Autodesk Fusion 360 part; units mm, degrees
note: some values were not read from the file. Chosen so that the rebuilt part matches the saved one: which face or edge a step refers to. Set by a fixed rule: which sketch regions a step uses.
(part 6 of 7)
  arc A131 (-37.243, 7.9658) -> (-36.8156, 8.2763) centre (-37.2058, 8.364) ccw
  spline S129 degree 3 poles (-38.191, 7.9821) (-37.7562, 8.0001) (-37.442, 7.9843) (-37.243, 7.9658) knots 0 0 0 0 1 1 1 1
  spline S130 degree 3 poles (-41.6177, 7.3659) (-40.1262, 7.8053) (-38.9736, 7.9493) (-38.191, 7.9821) knots 0 0 0 0 1 1 1 1
  arc A132 (-41.6177, 7.3659) -> (-41.857, 5.8552) centre (0, 0) ccw
  spline S131 degree 3 poles (-38.7884, 4.2102) (-39.5225, 4.4833) (-40.5743, 4.9764) (-41.857, 5.8552) knots 0 0 0 0 1 1 1 1
  spline S132 degree 3 poles (-37.8817, 3.9328) (-38.0767, 3.9767) (-38.3805, 4.0588) (-38.7884, 4.2102) knots 0 0 0 0 1 1 1 1
  arc A133 (-37.5712, 3.5054) -> (-37.8817, 3.9328) centre (-37.9695, 3.5426) ccw
  arc A134 (-37.5712, 3.5054) -> (-37.657, 2.4152) centre (0, 0) ccw
  arc A135 (-38.0306, 2.0416) -> (-37.657, 2.4152) centre (-38.0562, 2.4408) ccw
  spline S133 degree 3 poles (-38.9695, 1.9094) (-38.5429, 1.9952) (-38.23, 2.0288) (-38.0306, 2.0416) knots 0 0 0 0 1 1 1 1
  spline S134 degree 3 poles (-42.2576, 0.7648) (-40.8532, 1.4321) (-39.7373, 1.7546) (-38.9695, 1.9094) knots 0 0 0 0 1 1 1 1
  arc A136 (-42.2576, 0.7648) -> (-42.2576, -0.7648) centre (0, 0) ccw
  spline S135 degree 3 poles (-38.9695, -1.9094) (-39.7373, -1.7546) (-40.8532, -1.4321) (-42.2576, -0.7648) knots 0 0 0 0 1 1 1 1
  spline S136 degree 3 poles (-38.0306, -2.0416) (-38.23, -2.0288) (-38.5429, -1.9952) (-38.9695, -1.9094) knots 0 0 0 0 1 1 1 1
  arc A137 (-37.657, -2.4152) -> (-38.0306, -2.0416) centre (-38.0562, -2.4408) ccw
  arc A138 (-37.657, -2.4152) -> (-37.5712, -3.5054) centre (0, 0) ccw
  arc A139 (-37.8817, -3.9328) -> (-37.5712, -3.5054) centre (-37.9695, -3.5426) ccw
  spline S137 degree 3 poles (-38.7884, -4.2102) (-38.3805, -4.0588) (-38.0767, -3.9767) (-37.8817, -3.9328) knots 0 0 0 0 1 1 1 1
  spline S138 degree 3 poles (-41.857, -5.8552) (-40.5743, -4.9764) (-39.5225, -4.4833) (-38.7884, -4.2102) knots 0 0 0 0 1 1 1 1
  arc A140 (-41.857, -5.8552) -> (-41.6177, -7.3659) centre (0, 0) ccw
  spline S139 degree 3 poles (-38.191, -7.9821) (-38.9736, -7.9493) (-40.1262, -7.8053) (-41.6177, -7.3659) knots 0 0 0 0 1 1 1 1
  spline S140 degree 3 poles (-37.243, -7.9658) (-37.442, -7.9843) (-37.7562, -8.0001) (-38.191, -7.9821) knots 0 0 0 0 1 1 1 1
  arc A141 (-36.8156, -8.2763) -> (-37.243, -7.9658) centre (-37.2058, -8.364) ccw
  arc A142 (-36.8156, -8.2763) -> (-36.5603, -9.3397) centre (0, 0) ccw
  arc A143 (-36.8001, -9.8104) -> (-36.5603, -9.3397) centre (-36.9478, -9.4387) ccw
  spline S141 degree 3 poles (-37.6523, -10.2263) (-37.273, -10.0128) (-36.9859, -9.8842) (-36.8001, -9.8104) knots 0 0 0 0 1 1 1 1
  spline S142 degree 3 poles (-40.4257, -12.331) (-39.2962, -11.2623) (-38.3346, -10.6107) (-37.6523, -10.2263) knots 0 0 0 0 1 1 1 1
  arc A144 (-40.4257, -12.331) -> (-39.953, -13.7857) centre (0, 0) ccw
  spline S143 degree 3 poles (-36.4722, -13.8582) (-37.2502, -13.9482) (-38.4112, -13.9863) (-39.953, -13.7857) knots 0 0 0 0 1 1 1 1
  spline S144 degree 3 poles (-35.5383, -13.6938) (-35.732, -13.7432) (-36.0399, -13.808) (-36.4722, -13.8582) knots 0 0 0 0 1 1 1 1
  arc A145 (-35.0676, -13.9336) -> (-35.5383, -13.6938) centre (-35.4393, -14.0813) ccw
  arc A146 (-35.0676, -13.9336) -> (-34.6491, -14.944) centre (0, 0) ccw
  arc A147 (-34.8123, -15.4464) -> (-34.6491, -14.944) centre (-35.0164, -15.1024) ccw
  spline S145 degree 3 poles (-35.5889, -15.9905) (-35.2478, -15.7204) (-34.9843, -15.5484) (-34.8123, -15.4464) knots 0 0 0 0 1 1 1 1
  spline S146 degree 3 poles (-37.999, -18.5031) (-37.0506, -17.271) (-36.2028, -16.477) (-35.5889, -15.9905) knots 0 0 0 0 1 1 1 1
  arc A148 (-37.999, -18.5031) -> (-37.3046, -19.866) centre (0, 0) ccw
  spline S147 degree 3 poles (-33.8552, -19.3931) (-34.6096, -19.6037) (-35.7503, -19.823) (-37.3046, -19.866) knots 0 0 0 0 1 1 1 1
  spline S148 degree 3 poles (-32.9586, -19.0846) (-33.1422, -19.1638) (-33.4362, -19.2759) (-33.8552, -19.3931) knots 0 0 0 0 1 1 1 1
  arc A149 (-32.4562, -19.2479) -> (-32.9586, -19.0846) centre (-32.8002, -19.4519) ccw
  arc A150 (-32.4562, -19.2479) -> (-31.8848, -20.1803) centre (0, 0) ccw
  arc A151 (-31.9674, -20.7021) -> (-31.8848, -20.1803) centre (-32.2228, -20.3942) ccw
  spline S149 degree 3 poles (-32.6493, -21.3609) (-32.3546, -21.0408) (-32.1213, -20.8297) (-31.9674, -20.7021) knots 0 0 0 0 1 1 1 1
  spline S150 degree 3 poles (-34.6367, -24.2197) (-33.8927, -22.8543) (-33.1795, -21.9375) (-32.6493, -21.3609) knots 0 0 0 0 1 1 1 1
  arc A152 (-34.6367, -24.2197) -> (-33.7376, -25.4571) centre (0, 0) ccw
  spline S151 degree 3 poles (-30.4047, -24.4505) (-31.1168, -24.7765) (-32.2092, -25.1715) (-33.7376, -25.4571) knots 0 0 0 0 1 1 1 1
  spline S152 degree 3 poles (-29.5673, -24.0055) (-29.7363, -24.1124) (-30.0091, -24.2691) (-30.4047, -24.4505) knots 0 0 0 0 1 1 1 1
  arc A153 (-29.0455, -24.0882) -> (-29.5673, -24.0055) centre (-29.3534, -24.3435) ccw
  arc A154 (-29.0455, -24.0882) -> (-28.3353, -24.9197) centre (0, 0) ccw
  arc A155 (-28.3353, -25.448) -> (-28.3353, -24.9197) centre (-28.6357, -25.1839) ccw
  spline S153 degree 3 poles (-28.9058, -26.2054) (-28.6648, -25.8431) (-28.4673, -25.5981) (-28.3353, -25.448) knots 0 0 0 0 1 1 1 1
  spline S154 degree 3 poles (-30.4214, -29.3399) (-29.9002, -27.8749) (-29.3392, -26.8578) (-28.9058, -26.2054) knots 0 0 0 0 1 1 1 1
  arc A156 (-30.4214, -29.3399) -> (-29.3399, -30.4214) centre (0, 0) ccw
  spline S155 degree 3 poles (-26.2054, -28.9058) (-26.8578, -29.3392) (-27.8749, -29.9002) (-29.3399, -30.4214) knots 0 0 0 0 1 1 1 1
  spline S156 degree 3 poles (-25.448, -28.3353) (-25.5981, -28.4673) (-25.8431, -28.6648) (-26.2054, -28.9058) knots 0 0 0 0 1 1 1 1
  arc A157 (-24.9197, -28.3353) -> (-25.448, -28.3353) centre (-25.1839, -28.6357) ccw
  arc A158 (-24.9197, -28.3353) -> (-24.0882, -29.0455) centre (0, 0) ccw
  arc A159 (-24.0055, -29.5673) -> (-24.0882, -29.0455) centre (-24.3435, -29.3534) ccw
  spline S157 degree 3 poles (-24.4505, -30.4047) (-24.2691, -30.0091) (-24.1124, -29.7363) (-24.0055, -29.5673) knots 0 0 0 0 1 1 1 1
  spline S158 degree 3 poles (-25.4571, -33.7376) (-25.1715, -32.2092) (-24.7765, -31.1168) (-24.4505, -30.4047) knots 0 0 0 0 1 1 1 1
  arc A160 (-25.4571, -33.7376) -> (-24.2197, -34.6367) centre (0, 0) ccw
  spline S159 degree 3 poles (-21.3609, -32.6493) (-21.9375, -33.1795) (-22.8543, -33.8927) (-24.2197, -34.6367) knots 0 0 0 0 1 1 1 1
  circle A161 centre (0, 0) radius 3.85
extrude "Extrude2'''" add sketch "Sketch21" along normal blind -8 and the other way blind -40 separate body contours A0 A161 makes body 8 in component "Spur Gear (40 teeth)"
sketch "Sketch22" plane through (0, 20, 0) normal (0, 1, 0) x (-1, 0, 0)
  circle A0 centre (0, 0) radius 3.85
  circle A1 centre (58.2177, 14.5153) radius 5.25
  circle A2 centre (-41.6795, 43.1604) radius 5.25
  circle A3 centre (-16.5382, -57.6757) radius 5.25
  line L0 (-22.7416, -43.0299) -> (-27.9212, -61.0931)
  arc A4 (-27.9212, -61.0931) -> (-27.7213, -63.2604) centre (-25.0374, -61.9201) ccw
  arc A5 (-27.7213, -63.2604) -> (-10.0139, -68.3379) centre (-16.5382, -57.6757) ccw
  arc A6 (-10.0139, -68.3379) -> (-8.6959, -66.6059) centre (-11.5797, -65.779) ccw
  line L1 (-8.6959, -66.6059) -> (-3.5164, -48.5426)
  arc A7 (48.6358, 1.8201) -> (-3.5164, -48.5426) centre (66.1751, -68.5263) ccw
  line L2 (48.6358, 1.8201) -> (66.8688, 6.3661)
  arc A8 (66.8688, 6.3661) -> (68.6458, 7.6228) centre (66.143, 9.277) ccw
  arc A9 (68.6458, 7.6228) -> (64.1893, 25.4967) centre (58.2177, 14.5153) ccw
  arc A10 (64.1893, 25.4967) -> (62.0304, 25.772) centre (62.7561, 22.8612) ccw
  line L3 (62.0304, 25.772) -> (43.7973, 21.226)
  arc A11 (-25.8942, 41.2097) -> (43.7973, 21.226) centre (26.258, 91.5725) ccw
  line L4 (-25.8942, 41.2097) -> (-38.9476, 54.727)
  arc A12 (-38.9476, 54.727) -> (-40.9244, 55.6376) centre (-41.1056, 52.643) ccw
  arc A13 (-40.9244, 55.6376) -> (-54.1754, 42.8412) centre (-41.6795, 43.1604) ccw
  arc A14 (-54.1754, 42.8412) -> (-53.3344, 40.8338) centre (-51.1764, 42.9178) ccw
  line L5 (-53.3344, 40.8338) -> (-40.2809, 27.3166)
  arc A15 (-22.7416, -43.0299) -> (-40.2809, 27.3166) centre (-92.4331, -23.0462) ccw
  circle A16 centre (0, 0) radius 3.85
extrude "Extrude3'" add sketch "Sketch22" along normal blind 40 and the other way blind 8 contours A0 A16 bodies 6 in component "Component''"
sketch "Sketch23" plane through (0, 8, 0) normal (0, 1, 0) x (-1, 0, 0)
  spline S0 degree 3 poles (-79.7947, 19.9812) (-78.771, 20.1522) (-77.8517, 20.2559) (-77.0419, 20.3133) knots 0 0 0 0 1 1 1 1
  spline S1 degree 3 poles (-77.0419, 20.3133) (-76.8232, 20.3288) (-76.6126, 20.341) (-76.41, 20.3501) knots 0 0 0 0 1 1 1 1
  arc A0 (-76.41, 20.3501) -> (-76.0422, 20.6449) centre (-76.4282, 20.7497) ccw
  arc A1 (-75.6235, 22.1292) -> (-76.0422, 20.6449) centre (0, 0) ccw
  arc A2 (-75.6235, 22.1292) -> (-75.7832, 22.5728) centre (-76.0074, 22.2416) ccw
  spline S2 degree 3 poles (-75.7832, 22.5728) (-75.9511, 22.6864) (-76.1243, 22.8068) (-76.3027, 22.9343) knots 0 0 0 0 1 1 1 1
  spline S3 degree 3 poles (-76.3027, 22.9343) (-76.9632, 23.4064) (-77.6928, 23.9752) (-78.4763, 24.6558) knots 0 0 0 0 1 1 1 1
  arc A3 (-77.981, 26.1802) -> (-78.4763, 24.6558) centre (0, 0) ccw
  spline S4 degree 3 poles (-77.981, 26.1802) (-76.9471, 26.2704) (-76.0225, 26.3016) (-75.2107, 26.2953) knots 0 0 0 0 1 1 1 1
  spline S5 degree 3 poles (-75.2107, 26.2953) (-74.9914, 26.2937) (-74.7805, 26.2892) (-74.5778, 26.2825) knots 0 0 0 0 1 1 1 1
  arc A4 (-74.5778, 26.2825) -> (-74.188, 26.5475) centre (-74.5646, 26.6822) ccw
  arc A5 (-73.6542, 27.9944) -> (-74.188, 26.5475) centre (0, 0) ccw
  arc A6 (-73.6542, 27.9944) -> (-73.7785, 28.4491) centre (-74.0281, 28.1365) ccw
  spline S6 degree 3 poles (-73.7785, 28.4491) (-73.937, 28.5755) (-74.1003, 28.7092) (-74.2681, 28.8503) knots 0 0 0 0 1 1 1 1
  spline S7 degree 3 poles (-74.2681, 28.8503) (-74.8895, 29.3727) (-75.5723, 29.997) (-76.2999, 30.737) knots 0 0 0 0 1 1 1 1
  arc A7 (-75.6865, 32.2178) -> (-76.2999, 30.737) centre (0, 0) ccw
  spline S8 degree 3 poles (-75.6865, 32.2178) (-74.6487, 32.2266) (-73.7245, 32.1852) (-72.9157, 32.1152) knots 0 0 0 0 1 1 1 1
  spline S9 degree 3 poles (-72.9157, 32.1152) (-72.6972, 32.0964) (-72.4873, 32.0754) (-72.2858, 32.0528) knots 0 0 0 0 1 1 1 1
  arc A8 (-72.2858, 32.0528) -> (-71.8764, 32.2864) centre (-72.2413, 32.4503) ccw
  arc A9 (-71.2307, 33.6869) -> (-71.8764, 32.2864) centre (0, 0) ccw
  arc A10 (-71.2307, 33.6869) -> (-71.319, 34.15) centre (-71.5923, 33.8579) ccw
  spline S10 degree 3 poles (-71.319, 34.15) (-71.4671, 34.2885) (-71.6193, 34.4345) (-71.7756, 34.5883) knots 0 0 0 0 1 1 1 1
  spline S11 degree 3 poles (-71.7756, 34.5883) (-72.3541, 35.1579) (-72.9858, 35.8338) (-73.6531, 36.6287) knots 0 0 0 0 1 1 1 1
  arc A11 (-72.9254, 38.0568) -> (-73.6531, 36.6287) centre (0, 0) ccw
  spline S12 degree 3 poles (-72.9254, 38.0568) (-71.8901, 37.9841) (-70.972, 37.8704) (-70.1712, 37.7371) knots 0 0 0 0 1 1 1 1
  spline S13 degree 3 poles (-70.1712, 37.7371) (-69.9549, 37.7012) (-69.7473, 37.6638) (-69.5482, 37.6254) knots 0 0 0 0 1 1 1 1
  arc A12 (-69.5482, 37.6254) -> (-69.1217, 37.8262) centre (-69.4726, 38.0182) ccw
  arc A13 (-68.3681, 39.1718) -> (-69.1217, 37.8262) centre (0, 0) ccw
  arc A14 (-68.3681, 39.1718) -> (-68.4198, 39.6403) centre (-68.7152, 39.3706) ccw
  spline S14 degree 3 poles (-68.4198, 39.6403) (-68.5565, 39.79) (-68.6969, 39.9475) (-68.8406, 40.1132) knots 0 0 0 0 1 1 1 1
  spline S15 degree 3 poles (-68.8406, 40.1132) (-69.3726, 40.7264) (-69.9493, 41.4498) (-70.5522, 42.2945) knots 0 0 0 0 1 1 1 1
  arc A15 (-69.7147, 43.6612) -> (-70.5522, 42.2945) centre (0, 0) ccw
  spline S16 degree 3 poles (-69.7147, 43.6612) (-68.6883, 43.5075) (-67.7819, 43.322) (-66.9941, 43.1264) knots 0 0 0 0 1 1 1 1
  spline S17 degree 3 poles (-66.9941, 43.1264) (-66.7812, 43.0736) (-66.5772, 43.02) (-66.3817, 42.9661) knots 0 0 0 0 1 1 1 1
  arc A16 (-66.3817, 42.9661) -> (-65.9408, 43.1328) centre (-66.2755, 43.3518) ccw
  arc A17 (-65.084, 44.4151) -> (-65.9408, 43.1328) centre (0, 0) ccw
  arc A18 (-65.084, 44.4151) -> (-65.0987, 44.8863) centre (-65.4144, 44.6406) ccw
  spline S18 degree 3 poles (-65.0987, 44.8863) (-65.2233, 45.0463) (-65.3508, 45.2143) (-65.4811, 45.3907) knots 0 0 0 0 1 1 1 1
  spline S19 degree 3 poles (-65.4811, 45.3907) (-65.9633, 46.0437) (-66.4815, 46.8101) (-67.0163, 47.6996) knots 0 0 0 0 1 1 1 1
  arc A19 (-66.0742, 48.9963) -> (-67.0163, 47.6996) centre (0, 0) ccw
  spline S20 degree 3 poles (-66.0742, 48.9963) (-65.063, 48.7626) (-64.174, 48.5066) (-63.4039, 48.2497) knots 0 0 0 0 1 1 1 1
  spline S21 degree 3 poles (-63.4039, 48.2497) (-63.1959, 48.1804) (-62.9966, 48.111) (-62.806, 48.0419) knots 0 0 0 0 1 1 1 1
  arc A20 (-62.806, 48.0419) -> (-62.3533, 48.1735) centre (-62.6699, 48.418) ccw
  arc A21 (-61.3986, 49.3846) -> (-62.3533, 48.1735) centre (0, 0) ccw
  arc A22 (-61.3986, 49.3846) -> (-61.3763, 49.8555) centre (-61.7102, 49.6353) ccw
  spline S22 degree 3 poles (-61.3763, 49.8555) (-61.4879, 50.0247) (-61.6019, 50.2023) (-61.7179, 50.3883) knots 0 0 0 0 1 1 1 1
  spline S23 degree 3 poles (-61.7179, 50.3883) (-62.1475, 51.0772) (-62.6039, 51.8819) (-63.0673, 52.8106) knots 0 0 0 0 1 1 1 1
  arc A23 (-62.0263, 54.0294) -> (-63.0673, 52.8106) centre (0, 0) ccw
  spline S24 degree 3 poles (-62.0263, 54.0294) (-61.0366, 53.717) (-60.1704, 53.3921) (-59.4228, 53.0756) knots 0 0 0 0 1 1 1 1
  spline S25 degree 3 poles (-59.4228, 53.0756) (-59.2209, 52.9901) (-59.0277, 52.9053) (-58.8431, 52.8215) knots 0 0 0 0 1 1 1 1
  arc A24 (-58.8431, 52.8215) -> (-58.3815, 52.9172) centre (-58.6778, 53.1858) ccw
  arc A25 (-57.3346, 54.0497) -> (-58.3815, 52.9172) centre (0, 0) ccw
  arc A26 (-57.3346, 54.0497) -> (-57.2755, 54.5174) centre (-57.6257, 54.324) ccw
  spline S26 degree 3 poles (-57.2755, 54.5174) (-57.3735, 54.6948) (-57.4732, 54.8807) (-57.5742, 55.0753) knots 0 0 0 0 1 1 1 1
  spline S27 degree 3 poles (-57.5742, 55.0753) (-57.9484, 55.7958) (-58.3403, 56.6338) (-58.7294, 57.596) knots 0 0 0 0 1 1 1 1
  arc A27 (-57.596, 58.7294) -> (-58.7294, 57.596) centre (0, 0) ccw
  spline S28 degree 3 poles (-57.596, 58.7294) (-56.6338, 58.3403) (-55.7958, 57.9484) (-55.0753, 57.5742) knots 0 0 0 0 1 1 1 1
  spline S29 degree 3 poles (-55.0753, 57.5742) (-54.8807, 57.4732) (-54.6948, 57.3735) (-54.5174, 57.2755) knots 0 0 0 0 1 1 1 1
  arc A28 (-54.5174, 57.2755) -> (-54.0497, 57.3346) centre (-54.324, 57.6257) ccw
  arc A29 (-52.9172, 58.3815) -> (-54.0497, 57.3346) centre (0, 0) ccw
  arc A30 (-52.9172, 58.3815) -> (-52.8215, 58.8431) centre (-53.1858, 58.6778) ccw
  spline S30 degree 3 poles (-52.8215, 58.8431) (-52.9053, 59.0277) (-52.9901, 59.2209) (-53.0756, 59.4228) knots 0 0 0 0 1 1 1 1
  spline S31 degree 3 poles (-53.0756, 59.4228) (-53.3921, 60.1704) (-53.717, 61.0366) (-54.0294, 62.0263) knots 0 0 0 0 1 1 1 1
  arc A31 (-52.8106, 63.0673) -> (-54.0294, 62.0263) centre (0, 0) ccw
  spline S32 degree 3 poles (-52.8106, 63.0673) (-51.8819, 62.6039) (-51.0772, 62.1475) (-50.3883, 61.7179) knots 0 0 0 0 1 1 1 1
  spline S33 degree 3 poles (-50.3883, 61.7179) (-50.2023, 61.6019) (-50.0247, 61.4879) (-49.8555, 61.3763) knots 0 0 0 0 1 1 1 1
  arc A32 (-49.8555, 61.3763) -> (-49.3846, 61.3986) centre (-49.6353, 61.7102) ccw
  arc A33 (-48.1735, 62.3533) -> (-49.3846, 61.3986) centre (0, 0) ccw
  arc A34 (-48.1735, 62.3533) -> (-48.0419, 62.806) centre (-48.418, 62.6699) ccw
  spline S34 degree 3 poles (-48.0419, 62.806) (-48.111, 62.9966) (-48.1804, 63.1959) (-48.2497, 63.4039) knots 0 0 0 0 1 1 1 1
  spline S35 degree 3 poles (-48.2497, 63.4039) (-48.5066, 64.174) (-48.7626, 65.063) (-48.9963, 66.0742) knots 0 0 0 0 1 1 1 1
  arc A35 (-47.6996, 67.0163) -> (-48.9963, 66.0742) centre (0, 0) ccw
  spline S36 degree 3 poles (-47.6996, 67.0163) (-46.8101, 66.4815) (-46.0437, 65.9633) (-45.3907, 65.4811) knots 0 0 0 0 1 1 1 1
  spline S37 degree 3 poles (-45.3907, 65.4811) (-45.2143, 65.3508) (-45.0463, 65.2233) (-44.8863, 65.0987) knots 0 0 0 0 1 1 1 1
  arc A36 (-44.8863, 65.0987) -> (-44.4151, 65.084) centre (-44.6406, 65.4144) ccw
  arc A37 (-43.1328, 65.9408) -> (-44.4151, 65.084) centre (0, 0) ccw
  arc A38 (-43.1328, 65.9408) -> (-42.9661, 66.3817) centre (-43.3518, 66.2755) ccw
  spline S38 degree 3 poles (-42.9661, 66.3817) (-43.02, 66.5772) (-43.0736, 66.7812) (-43.1264, 66.9941) knots 0 0 0 0 1 1 1 1
  spline S39 degree 3 poles (-43.1264, 66.9941) (-43.322, 67.7819) (-43.5075, 68.6883) (-43.6612, 69.7147) knots 0 0 0 0 1 1 1 1
  arc A39 (-42.2945, 70.5522) -> (-43.6612, 69.7147) centre (0, 0) ccw
  spline S40 degree 3 poles (-42.2945, 70.5522) (-41.4498, 69.9493) (-40.7264, 69.3726) (-40.1132, 68.8406) knots 0 0 0 0 1 1 1 1
  spline S41 degree 3 poles (-40.1132, 68.8406) (-39.9475, 68.6969) (-39.79, 68.5565) (-39.6403, 68.4198) knots 0 0 0 0 1 1 1 1
  arc A40 (-39.6403, 68.4198) -> (-39.1718, 68.3681) centre (-39.3706, 68.7152) ccw
  arc A41 (-37.8262, 69.1217) -> (-39.1718, 68.3681) centre (0, 0) ccw
  arc A42 (-37.8262, 69.1217) -> (-37.6254, 69.5482) centre (-38.0182, 69.4726) ccw
  spline S42 degree 3 poles (-37.6254, 69.5482) (-37.6638, 69.7473) (-37.7012, 69.9549) (-37.7371, 70.1712) knots 0 0 0 0 1 1 1 1
  spline S43 degree 3 poles (-37.7371, 70.1712) (-37.8704, 70.972) (-37.9841, 71.8901) (-38.0568, 72.9254) knots 0 0 0 0 1 1 1 1
  arc A43 (-36.6287, 73.6531) -> (-38.0568, 72.9254) centre (0, 0) ccw
  spline S44 degree 3 poles (-36.6287, 73.6531) (-35.8338, 72.9858) (-35.1579, 72.3541) (-34.5883, 71.7756) knots 0 0 0 0 1 1 1 1
  spline S45 degree 3 poles (-34.5883, 71.7756) (-34.4345, 71.6193) (-34.2885, 71.4671) (-34.15, 71.319) knots 0 0 0 0 1 1 1 1
  arc A44 (-34.15, 71.319) -> (-33.6869, 71.2307) centre (-33.8579, 71.5923) ccw
  arc A45 (-32.2864, 71.8764) -> (-33.6869, 71.2307) centre (0, 0) ccw
  arc A46 (-32.2864, 71.8764) -> (-32.0528, 72.2858) centre (-32.4503, 72.2413) ccw
  spline S46 degree 3 poles (-32.0528, 72.2858) (-32.0754, 72.4873) (-32.0964, 72.6972) (-32.1152, 72.9157) knots 0 0 0 0 1 1 1 1
  spline S47 degree 3 poles (-32.1152, 72.9157) (-32.1852, 73.7245) (-32.2266, 74.6487) (-32.2178, 75.6865) knots 0 0 0 0 1 1 1 1
  arc A47 (-30.737, 76.2999) -> (-32.2178, 75.6865) centre (0, 0) ccw
  spline S48 degree 3 poles (-30.737, 76.2999) (-29.997, 75.5723) (-29.3727, 74.8895) (-28.8503, 74.2681) knots 0 0 0 0 1 1 1 1
  spline S49 degree 3 poles (-28.8503, 74.2681) (-28.7092, 74.1003) (-28.5755, 73.937) (-28.4491, 73.7785) knots 0 0 0 0 1 1 1 1
  arc A48 (-28.4491, 73.7785) -> (-27.9944, 73.6542) centre (-28.1365, 74.0281) ccw
  arc A49 (-26.5475, 74.188) -> (-27.9944, 73.6542) centre (0, 0) ccw
  arc A50 (-26.5475, 74.188) -> (-26.2825, 74.5778) centre (-26.6822, 74.5646) ccw
  spline S50 degree 3 poles (-26.2825, 74.5778) (-26.2892, 74.7805) (-26.2937, 74.9914) (-26.2953, 75.2107) knots 0 0 0 0 1 1 1 1
  spline S51 degree 3 poles (-26.2953, 75.2107) (-26.3016, 76.0225) (-26.2704, 76.9471) (-26.1802, 77.981) knots 0 0 0 0 1 1 1 1
  arc A51 (-24.6558, 78.4763) -> (-26.1802, 77.981) centre (0, 0) ccw
  spline S52 degree 3 poles (-24.6558, 78.4763) (-23.9752, 77.6928) (-23.4064, 76.9632) (-22.9343, 76.3027) knots 0 0 0 0 1 1 1 1
  spline S53 degree 3 poles (-22.9343, 76.3027) (-22.8068, 76.1243) (-22.6864, 75.9511) (-22.5728, 75.7832) knots 0 0 0 0 1 1 1 1
  arc A52 (-22.5728, 75.7832) -> (-22.1292, 75.6235) centre (-22.2416, 76.0074) ccw
  arc A53 (-20.6449, 76.0422) -> (-22.1292, 75.6235) centre (0, 0) ccw
  arc A54 (-20.6449, 76.0422) -> (-20.3501, 76.41) centre (-20.7497, 76.4282) ccw
  spline S54 degree 3 poles (-20.3501, 76.41) (-20.341, 76.6126) (-20.3288, 76.8232) (-20.3133, 77.0419) knots 0 0 0 0 1 1 1 1
  spline S55 degree 3 poles (-20.3133, 77.0419) (-20.2559, 77.8517) (-20.1522, 78.771) (-19.9812, 79.7947) knots 0 0 0 0 1 1 1 1
  arc A55 (-18.4227, 80.1689) -> (-19.9812, 79.7947) centre (0, 0) ccw
  spline S56 degree 3 poles (-18.4227, 80.1689) (-17.8055, 79.3344) (-17.2958, 78.5624) (-16.877, 77.8669) knots 0 0 0 0 1 1 1 1
  spline S57 degree 3 poles (-16.877, 77.8669) (-16.7639, 77.6791) (-16.6574, 77.4969) (-16.5573, 77.3206) knots 0 0 0 0 1 1 1 1
  arc A56 (-16.5573, 77.3206) -> (-16.1277, 77.1267) centre (-16.2095, 77.5182) ccw
  arc A57 (-14.6151, 77.4275) -> (-16.1277, 77.1267) centre (0, 0) ccw
  arc A58 (-14.6151, 77.4275) -> (-14.2923, 77.7712) centre (-14.6893, 77.8206) ccw
  spline S58 degree 3 poles (-14.2923, 77.7712) (-14.2673, 77.9723) (-14.2387, 78.1814) (-14.2061, 78.3982) knots 0 0 0 0 1 1 1 1
  spline S59 degree 3 poles (-14.2061, 78.3982) (-14.0853, 79.201) (-13.9098, 80.1093) (-13.659, 81.1164) knots 0 0 0 0 1 1 1 1
  arc A59 (-12.0759, 81.3672) -> (-13.659, 81.1164) centre (0, 0) ccw
  spline S60 degree 3 poles (-12.0759, 81.3672) (-11.5261, 80.4868) (-11.0785, 79.6772) (-10.7156, 78.951) knots 0 0 0 0 1 1 1 1
  spline S61 degree 3 poles (-10.7156, 78.951) (-10.6176, 78.7549) (-10.5258, 78.5649) (-10.4398, 78.3813) knots 0 0 0 0 1 1 1 1
  arc A60 (-10.4398, 78.3813) -> (-10.0267, 78.1543) centre (-10.0776, 78.551) ccw
  arc A61 (-8.4951, 78.3355) -> (-10.0267, 78.1543) centre (0, 0) ccw
  arc A62 (-8.4951, 78.3355) -> (-8.1464, 78.6528) centre (-8.5383, 78.7332) ccw
  spline S62 degree 3 poles (-8.1464, 78.6528) (-8.1057, 78.8514) (-8.0608, 79.0575) (-8.0112, 79.2711) knots 0 0 0 0 1 1 1 1
  spline S63 degree 3 poles (-8.0112, 79.2711) (-7.8278, 80.0619) (-7.5816, 80.9537) (-7.2526, 81.938) knots 0 0 0 0 1 1 1 1
  arc A63 (-5.6547, 82.0638) -> (-7.2526, 81.938) centre (0, 0) ccw
  spline S64 degree 3 poles (-5.6547, 82.0638) (-5.1757, 81.1431) (-4.793, 80.3008) (-4.4881, 79.5484) knots 0 0 0 0 1 1 1 1
  spline S65 degree 3 poles (-4.4881, 79.5484) (-4.4058, 79.3452) (-4.3292, 79.1486) (-4.2579, 78.9588) knots 0 0 0 0 1 1 1 1
  arc A64 (-4.2579, 78.9588) -> (-3.8638, 78.7) centre (-3.8835, 79.0995) ccw
  arc A65 (-2.3228, 78.7606) -> (-3.8638, 78.7) centre (0, 0) ccw
  arc A66 (-2.3228, 78.7606) -> (-1.9503, 79.0495) centre (-2.3346, 79.1604) ccw
  spline S66 degree 3 poles (-1.9503, 79.0495) (-1.8941, 79.2443) (-1.8331, 79.4462) (-1.767, 79.6553) knots 0 0 0 0 1 1 1 1
  spline S67 degree 3 poles (-1.767, 79.6553) (-1.5221, 80.4293) (-1.2067, 81.299) (-0.8014, 82.2545) knots 0 0 0 0 1 1 1 1
  arc A67 (0.8014, 82.2545) -> (-0.8014, 82.2545) centre (0, 0) ccw
  spline S68 degree 3 poles (0.8014, 82.2545) (1.2067, 81.299) (1.5221, 80.4293) (1.767, 79.6553) knots 0 0 0 0 1 1 1 1
  spline S69 degree 3 poles (1.767, 79.6553) (1.8331, 79.4462) (1.8941, 79.2443) (1.9503, 79.0495) knots 0 0 0 0 1 1 1 1
  arc A68 (1.9503, 79.0495) -> (2.3228, 78.7606) centre (2.3346, 79.1604) ccw
  arc A69 (3.8638, 78.7) -> (2.3228, 78.7606) centre (0, 0) ccw
  arc A70 (3.8638, 78.7) -> (4.2579, 78.9588) centre (3.8835, 79.0995) ccw
  spline S70 degree 3 poles (4.2579, 78.9588) (4.3292, 79.1486) (4.4058, 79.3452) (4.4881, 79.5484) knots 0 0 0 0 1 1 1 1
  spline S71 degree 3 poles (4.4881, 79.5484) (4.793, 80.3008) (5.1757, 81.1431) (5.6547, 82.0638) knots 0 0 0 0 1 1 1 1
  arc A71 (7.2526, 81.938) -> (5.6547, 82.0638) centre (0, 0) ccw
  spline S72 degree 3 poles (7.2526, 81.938) (7.5816, 80.9537) (7.8278, 80.0619) (8.0112, 79.2711) knots 0 0 0 0 1 1 1 1
  spline S73 degree 3 poles (8.0112, 79.2711) (8.0608, 79.0575) (8.1057, 78.8514) (8.1464, 78.6528) knots 0 0 0 0 1 1 1 1
  arc A72 (8.1464, 78.6528) -> (8.4951, 78.3355) centre (8.5383, 78.7332) ccw
  arc A73 (10.0267, 78.1543) -> (8.4951, 78.3355) centre (0, 0) ccw
  arc A74 (10.0267, 78.1543) -> (10.4398, 78.3813) centre (10.0776, 78.551) ccw
  spline S74 degree 3 poles (10.4398, 78.3813) (10.5258, 78.5649) (10.6176, 78.7549) (10.7156, 78.951) knots 0 0 0 0 1 1 1 1
  spline S75 degree 3 poles (10.7156, 78.951) (11.0785, 79.6772) (11.5261, 80.4868) (12.0759, 81.3672) knots 0 0 0 0 1 1 1 1
  arc A75 (13.659, 81.1164) -> (12.0759, 81.3672) centre (0, 0) ccw
  spline S76 degree 3 poles (13.659, 81.1164) (13.9098, 80.1093) (14.0853, 79.201) (14.2061, 78.3982) knots 0 0 0 0 1 1 1 1
  spline S77 degree 3 poles (14.2061, 78.3982) (14.2387, 78.1814) (14.2673, 77.9723) (14.2923, 77.7712) knots 0 0 0 0 1 1 1 1
  arc A76 (14.2923, 77.7712) -> (14.6151, 77.4275) centre (14.6893, 77.8206) ccw
  arc A77 (16.1277, 77.1267) -> (14.6151, 77.4275) centre (0, 0) ccw
  arc A78 (16.1277, 77.1267) -> (16.5573, 77.3206) centre (16.2095, 77.5182) ccw
  spline S78 degree 3 poles (16.5573, 77.3206) (16.6574, 77.4969) (16.7639, 77.6791) (16.877, 77.8669) knots 0 0 0 0 1 1 1 1
  spline S79 degree 3 poles (16.877, 77.8669) (17.2958, 78.5624) (17.8055, 79.3344) (18.4227, 80.1689) knots 0 0 0 0 1 1 1 1
  arc A79 (19.9812, 79.7947) -> (18.4227, 80.1689) centre (0, 0) ccw
  spline S80 degree 3 poles (19.9812, 79.7947) (20.1522, 78.771) (20.2559, 77.8517) (20.3133, 77.0419) knots 0 0 0 0 1 1 1 1
  spline S81 degree 3 poles (20.3133, 77.0419) (20.3288, 76.8232) (20.341, 76.6126) (20.3501, 76.41) knots 0 0 0 0 1 1 1 1
  arc A80 (20.3501, 76.41) -> (20.6449, 76.0422) centre (20.7497, 76.4282) ccw
  arc A81 (22.1292, 75.6235) -> (20.6449, 76.0422) centre (0, 0) ccw
  arc A82 (22.1292, 75.6235) -> (22.5728, 75.7832) centre (22.2416, 76.0074) ccw
  spline S82 degree 3 poles (22.5728, 75.7832) (22.6864, 75.9511) (22.8068, 76.1243) (22.9343, 76.3027) knots 0 0 0 0 1 1 1 1
  spline S83 degree 3 poles (22.9343, 76.3027) (23.4064, 76.9632) (23.9752, 77.6928) (24.6558, 78.4763) knots 0 0 0 0 1 1 1 1
  arc A83 (26.1802, 77.981) -> (24.6558, 78.4763) centre (0, 0) ccw
  spline S84 degree 3 poles (26.1802, 77.981) (26.2704, 76.9471) (26.3016, 76.0225) (26.2953, 75.2107) knots 0 0 0 0 1 1 1 1
  spline S85 degree 3 poles (26.2953, 75.2107) (26.2937, 74.9914) (26.2892, 74.7805) (26.2825, 74.5778) knots 0 0 0 0 1 1 1 1
  arc A84 (26.2825, 74.5778) -> (26.5475, 74.188) centre (26.6822, 74.5646) ccw
  arc A85 (27.9944, 73.6542) -> (26.5475, 74.188) centre (0, 0) ccw
  arc A86 (27.9944, 73.6542) -> (28.4491, 73.7785) centre (28.1365, 74.0281) ccw
  spline S86 degree 3 poles (28.4491, 73.7785) (28.5755, 73.937) (28.7092, 74.1003) (28.8503, 74.2681) knots 0 0 0 0 1 1 1 1
  spline S87 degree 3 poles (28.8503, 74.2681) (29.3727, 74.8895) (29.997, 75.5723) (30.737, 76.2999) knots 0 0 0 0 1 1 1 1
  arc A87 (32.2178, 75.6865) -> (30.737, 76.2999) centre (0, 0) ccw
  spline S88 degree 3 poles (32.2178, 75.6865) (32.2266, 74.6487) (32.1852, 73.7245) (32.1152, 72.9157) knots 0 0 0 0 1 1 1 1
  spline S89 degree 3 poles (32.1152, 72.9157) (32.0964, 72.6972) (32.0754, 72.4873) (32.0528, 72.2858) knots 0 0 0 0 1 1 1 1
  arc A88 (32.0528, 72.2858) -> (32.2864, 71.8764) centre (32.4503, 72.2413) ccw
  arc A89 (33.6869, 71.2307) -> (32.2864, 71.8764) centre (0, 0) ccw
  arc A90 (33.6869, 71.2307) -> (34.15, 71.319) centre (33.8579, 71.5923) ccw
  spline S90 degree 3 poles (34.15, 71.319) (34.2885, 71.4671) (34.4345, 71.6193) (34.5883, 71.7756) knots 0 0 0 0 1 1 1 1
  spline S91 degree 3 poles (34.5883, 71.7756) (35.1579, 72.3541) (35.8338, 72.9858) (36.6287, 73.6531) knots 0 0 0 0 1 1 1 1
  arc A91 (38.0568, 72.9254) -> (36.6287, 73.6531) centre (0, 0) ccw
  spline S92 degree 3 poles (38.0568, 72.9254) (37.9841, 71.8901) (37.8704, 70.972) (37.7371, 70.1712) knots 0 0 0 0 1 1 1 1
  spline S93 degree 3 poles (37.7371, 70.1712) (37.7012, 69.9549) (37.6638, 69.7473) (37.6254, 69.5482) knots 0 0 0 0 1 1 1 1
  arc A92 (37.6254, 69.5482) -> (37.8262, 69.1217) centre (38.0182, 69.4726) ccw
  arc A93 (39.1718, 68.3681) -> (37.8262, 69.1217) centre (0, 0) ccw
  arc A94 (39.1718, 68.3681) -> (39.6403, 68.4198) centre (39.3706, 68.7152) ccw
  spline S94 degree 3 poles (39.6403, 68.4198) (39.79, 68.5565) (39.9475, 68.6969) (40.1132, 68.8406) knots 0 0 0 0 1 1 1 1
  spline S95 degree 3 poles (40.1132, 68.8406) (40.7264, 69.3726) (41.4498, 69.9493) (42.2945, 70.5522) knots 0 0 0 0 1 1 1 1
  arc A95 (43.6612, 69.7147) -> (42.2945, 70.5522) centre (0, 0) ccw
  spline S96 degree 3 poles (43.6612, 69.7147) (43.5075, 68.6883) (43.322, 67.7819) (43.1264, 66.9941) knots 0 0 0 0 1 1 1 1
  spline S97 degree 3 poles (43.1264, 66.9941) (43.0736, 66.7812) (43.02, 66.5772) (42.9661, 66.3817) knots 0 0 0 0 1 1 1 1
  arc A96 (42.9661, 66.3817) -> (43.1328, 65.9408) centre (43.3518, 66.2755) ccw
  arc A97 (44.4151, 65.084) -> (43.1328, 65.9408) centre (0, 0) ccw
  arc A98 (44.4151, 65.084) -> (44.8863, 65.0987) centre (44.6406, 65.4144) ccw
  spline S98 degree 3 poles (44.8863, 65.0987) (45.0463, 65.2233) (45.2143, 65.3508) (45.3907, 65.4811) knots 0 0 0 0 1 1 1 1
  spline S99 degree 3 poles (45.3907, 65.4811) (46.0437, 65.9633) (46.8101, 66.4815) (47.6996, 67.0163) knots 0 0 0 0 1 1 1 1
  arc A99 (48.9963, 66.0742) -> (47.6996, 67.0163) centre (0, 0) ccw
  spline S100 degree 3 poles (48.9963, 66.0742) (48.7626, 65.063) (48.5066, 64.174) (48.2497, 63.4039) knots 0 0 0 0 1 1 1 1
  spline S101 degree 3 poles (48.2497, 63.4039) (48.1804, 63.1959) (48.111, 62.9966) (48.0419, 62.806) knots 0 0 0 0 1 1 1 1
  arc A100 (48.0419, 62.806) -> (48.1735, 62.3533) centre (48.418, 62.6699) ccw
  arc A101 (49.3846, 61.3986) -> (48.1735, 62.3533) centre (0, 0) ccw
  arc A102 (49.3846, 61.3986) -> (49.8555, 61.3763) centre (49.6353, 61.7102) ccw
  spline S102 degree 3 poles (49.8555, 61.3763) (50.0247, 61.4879) (50.2023, 61.6019) (50.3883, 61.7179) knots 0 0 0 0 1 1 1 1
  spline S103 degree 3 poles (50.3883, 61.7179) (51.0772, 62.1475) (51.8819, 62.6039) (52.8106, 63.0673) knots 0 0 0 0 1 1 1 1
  arc A103 (54.0294, 62.0263) -> (52.8106, 63.0673) centre (0, 0) ccw
  spline S104 degree 3 poles (54.0294, 62.0263) (53.717, 61.0366) (53.3921, 60.1704) (53.0756, 59.4228) knots 0 0 0 0 1 1 1 1
  spline S105 degree 3 poles (53.0756, 59.4228) (52.9901, 59.2209) (52.9053, 59.0277) (52.8215, 58.8431) knots 0 0 0 0 1 1 1 1
  arc A104 (52.8215, 58.8431) -> (52.9172, 58.3815) centre (53.1858, 58.6778) ccw
  arc A105 (54.0497, 57.3346) -> (52.9172, 58.3815) centre (0, 0) ccw
  arc A106 (54.0497, 57.3346) -> (54.5174, 57.2755) centre (54.324, 57.6257) ccw
  spline S106 degree 3 poles (54.5174, 57.2755) (54.6948, 57.3735) (54.8807, 57.4732) (55.0753, 57.5742) knots 0 0 0 0 1 1 1 1
  spline S107 degree 3 poles (55.0753, 57.5742) (55.7958, 57.9484) (56.6338, 58.3403) (57.596, 58.7294) knots 0 0 0 0 1 1 1 1
  arc A107 (58.7294, 57.596) -> (57.596, 58.7294) centre (0, 0) ccw
  spline S108 degree 3 poles (58.7294, 57.596) (58.3403, 56.6338) (57.9484, 55.7958) (57.5742, 55.0753) knots 0 0 0 0 1 1 1 1
  spline S109 degree 3 poles (57.5742, 55.0753) (57.4732, 54.8807) (57.3735, 54.6948) (57.2755, 54.5174) knots 0 0 0 0 1 1 1 1
  arc A108 (57.2755, 54.5174) -> (57.3346, 54.0497) centre (57.6257, 54.324) ccw
  arc A109 (58.3815, 52.9172) -> (57.3346, 54.0497) centre (0, 0) ccw
  arc A110 (58.3815, 52.9172) -> (58.8431, 52.8215) centre (58.6778, 53.1858) ccw
  spline S110 degree 3 poles (58.8431, 52.8215) (59.0277, 52.9053) (59.2209, 52.9901) (59.4228, 53.0756) knots 0 0 0 0 1 1 1 1
  spline S111 degree 3 poles (59.4228, 53.0756) (60.1704, 53.3921) (61.0366, 53.717) (62.0263, 54.0294) knots 0 0 0 0 1 1 1 1
  arc A111 (63.0673, 52.8106) -> (62.0263, 54.0294) centre (0, 0) ccw
  spline S112 degree 3 poles (63.0673, 52.8106) (62.6039, 51.8819) (62.1475, 51.0772) (61.7179, 50.3883) knots 0 0 0 0 1 1 1 1
  spline S113 degree 3 poles (61.7179, 50.3883) (61.6019, 50.2023) (61.4879, 50.0247) (61.3763, 49.8555) knots 0 0 0 0 1 1 1 1
  arc A112 (61.3763, 49.8555) -> (61.3986, 49.3846) centre (61.7102, 49.6353) ccw
  arc A113 (62.3533, 48.1735) -> (61.3986, 49.3846) centre (0, 0) ccw
  arc A114 (62.3533, 48.1735) -> (62.806, 48.0419) centre (62.6699, 48.418) ccw
  spline S114 degree 3 poles (62.806, 48.0419) (62.9966, 48.111) (63.1959, 48.1804) (63.4039, 48.2497) knots 0 0 0 0 1 1 1 1
  spline S115 degree 3 poles (63.4039, 48.2497) (64.174, 48.5066) (65.063, 48.7626) (66.0742, 48.9963) knots 0 0 0 0 1 1 1 1
  arc A115 (67.0163, 47.6996) -> (66.0742, 48.9963) centre (0, 0) ccw
  spline S116 degree 3 poles (67.0163, 47.6996) (66.4815, 46.8101) (65.9633, 46.0437) (65.4811, 45.3907) knots 0 0 0 0 1 1 1 1
  spline S117 degree 3 poles (65.4811, 45.3907) (65.3508, 45.2143) (65.2233, 45.0463) (65.0987, 44.8863) knots 0 0 0 0 1 1 1 1
  arc A116 (65.0987, 44.8863) -> (65.084, 44.4151) centre (65.4144, 44.6406) ccw
  arc A117 (65.9408, 43.1328) -> (65.084, 44.4151) centre (0, 0) ccw
  arc A118 (65.9408, 43.1328) -> (66.3817, 42.9661) centre (66.2755, 43.3518) ccw
  spline S118 degree 3 poles (66.3817, 42.9661) (66.5772, 43.02) (66.7812, 43.0736) (66.9941, 43.1264) knots 0 0 0 0 1 1 1 1
  spline S119 degree 3 poles (66.9941, 43.1264) (67.7819, 43.322) (68.6883, 43.5075) (69.7147, 43.6612) knots 0 0 0 0 1 1 1 1
  arc A119 (70.5522, 42.2945) -> (69.7147, 43.6612) centre (0, 0) ccw
  spline S120 degree 3 poles (70.5522, 42.2945) (69.9493, 41.4498) (69.3726, 40.7264) (68.8406, 40.1132) knots 0 0 0 0 1 1 1 1
  spline S121 degree 3 poles (68.8406, 40.1132) (68.6969, 39.9475) (68.5565, 39.79) (68.4198, 39.6403) knots 0 0 0 0 1 1 1 1
  arc A120 (68.4198, 39.6403) -> (68.3681, 39.1718) centre (68.7152, 39.3706) ccw
  arc A121 (69.1217, 37.8262) -> (68.3681, 39.1718) centre (0, 0) ccw
  arc A122 (69.1217, 37.8262) -> (69.5482, 37.6254) centre (69.4726, 38.0182) ccw
  spline S122 degree 3 poles (69.5482, 37.6254) (69.7473, 37.6638) (69.9549, 37.7012) (70.1712, 37.7371) knots 0 0 0 0 1 1 1 1
  spline S123 degree 3 poles (70.1712, 37.7371) (70.972, 37.8704) (71.8901, 37.9841) (72.9254, 38.0568) knots 0 0 0 0 1 1 1 1
  arc A123 (73.6531, 36.6287) -> (72.9254, 38.0568) centre (0, 0) ccw
  spline S124 degree 3 poles (73.6531, 36.6287) (72.9858, 35.8338) (72.3541, 35.1579) (71.7756, 34.5883) knots 0 0 0 0 1 1 1 1
  spline S125 degree 3 poles (71.7756, 34.5883) (71.6193, 34.4345) (71.4671, 34.2885) (71.319, 34.15) knots 0 0 0 0 1 1 1 1
  arc A124 (71.319, 34.15) -> (71.2307, 33.6869) centre (71.5923, 33.8579) ccw
  arc A125 (71.8764, 32.2864) -> (71.2307, 33.6869) centre (0, 0) ccw
  arc A126 (71.8764, 32.2864) -> (72.2858, 32.0528) centre (72.2413, 32.4503) ccw
  spline S126 degree 3 poles (72.2858, 32.0528) (72.4873, 32.0754) (72.6972, 32.0964) (72.9157, 32.1152) knots 0 0 0 0 1 1 1 1
  spline S127 degree 3 poles (72.9157, 32.1152) (73.7245, 32.1852) (74.6487, 32.2266) (75.6865, 32.2178) knots 0 0 0 0 1 1 1 1
  arc A127 (76.2999, 30.737) -> (75.6865, 32.2178) centre (0, 0) ccw
  spline S128 degree 3 poles (76.2999, 30.737) (75.5723, 29.997) (74.8895, 29.3727) (74.2681, 28.8503) knots 0 0 0 0 1 1 1 1
  spline S129 degree 3 poles (74.2681, 28.8503) (74.1003, 28.7092) (73.937, 28.5755) (73.7785, 28.4491) knots 0 0 0 0 1 1 1 1
  arc A128 (73.7785, 28.4491) -> (73.6542, 27.9944) centre (74.0281, 28.1365) ccw
  arc A129 (74.188, 26.5475) -> (73.6542, 27.9944) centre (0, 0) ccw
  arc A130 (74.188, 26.5475) -> (74.5778, 26.2825) centre (74.5646, 26.6822) ccw
  spline S130 degree 3 poles (74.5778, 26.2825) (74.7805, 26.2892) (74.9914, 26.2937) (75.2107, 26.2953) knots 0 0 0 0 1 1 1 1
  spline S131 degree 3 poles (75.2107, 26.2953) (76.0225, 26.3016) (76.9471, 26.2704) (77.981, 26.1802) knots 0 0 0 0 1 1 1 1
  arc A131 (78.4763, 24.6558) -> (77.981, 26.1802) centre (0, 0) ccw
  spline S132 degree 3 poles (78.4763, 24.6558) (77.6928, 23.9752) (76.9632, 23.4064) (76.3027, 22.9343) knots 0 0 0 0 1 1 1 1
  spline S133 degree 3 poles (76.3027, 22.9343) (76.1243, 22.8068) (75.9511, 22.6864) (75.7832, 22.5728) knots 0 0 0 0 1 1 1 1
  arc A132 (75.7832, 22.5728) -> (75.6235, 22.1292) centre (76.0074, 22.2416) ccw
  arc A133 (76.0422, 20.6449) -> (75.6235, 22.1292) centre (0, 0) ccw
  arc A134 (76.0422, 20.6449) -> (76.41, 20.3501) centre (76.4282, 20.7497) ccw
  spline S134 degree 3 poles (76.41, 20.3501) (76.6126, 20.341) (76.8232, 20.3288) (77.0419, 20.3133) knots 0 0 0 0 1 1 1 1
  spline S135 degree 3 poles (77.0419, 20.3133) (77.8517, 20.2559) (78.771, 20.1522) (79.7947, 19.9812) knots 0 0 0 0 1 1 1 1
  arc A135 (80.1689, 18.4227) -> (79.7947, 19.9812) centre (0, 0) ccw
  spline S136 degree 3 poles (80.1689, 18.4227) (79.3344, 17.8055) (78.5624, 17.2958) (77.8669, 16.877) knots 0 0 0 0 1 1 1 1
  spline S137 degree 3 poles (77.8669, 16.877) (77.6791, 16.7639) (77.4969, 16.6574) (77.3206, 16.5573) knots 0 0 0 0 1 1 1 1
  arc A136 (77.3206, 16.5573) -> (77.1267, 16.1277) centre (77.5182, 16.2095) ccw
  arc A137 (77.4275, 14.6151) -> (77.1267, 16.1277) centre (0, 0) ccw
  arc A138 (77.4275, 14.6151) -> (77.7712, 14.2923) centre (77.8206, 14.6893) ccw
  spline S138 degree 3 poles (77.7712, 14.2923) (77.9723, 14.2673) (78.1814, 14.2387) (78.3982, 14.2061) knots 0 0 0 0 1 1 1 1
  spline S139 degree 3 poles (78.3982, 14.2061) (79.201, 14.0853) (80.1093, 13.9098) (81.1164, 13.659) knots 0 0 0 0 1 1 1 1
  arc A139 (81.3672, 12.0759) -> (81.1164, 13.659) centre (0, 0) ccw
  spline S140 degree 3 poles (81.3672, 12.0759) (80.4868, 11.5261) (79.6772, 11.0785) (78.951, 10.7156) knots 0 0 0 0 1 1 1 1
  spline S141 degree 3 poles (78.951, 10.7156) (78.7549, 10.6176) (78.5649, 10.5258) (78.3813, 10.4398) knots 0 0 0 0 1 1 1 1
  arc A140 (78.3813, 10.4398) -> (78.1543, 10.0267) centre (78.551, 10.0776) ccw
  arc A141 (78.3355, 8.4951) -> (78.1543, 10.0267) centre (0, 0) ccw
  arc A142 (78.3355, 8.4951) -> (78.6528, 8.1464) centre (78.7332, 8.5383) ccw
  spline S142 degree 3 poles (78.6528, 8.1464) (78.8514, 8.1057) (79.0575, 8.0608) (79.2711, 8.0112) knots 0 0 0 0 1 1 1 1
  spline S143 degree 3 poles (79.2711, 8.0112) (80.0619, 7.8278) (80.9537, 7.5816) (81.938, 7.2526) knots 0 0 0 0 1 1 1 1
  arc A143 (82.0638, 5.6547) -> (81.938, 7.2526) centre (0, 0) ccw
  spline S144 degree 3 poles (82.0638, 5.6547) (81.1431, 5.1757) (80.3008, 4.793) (79.5484, 4.4881) knots 0 0 0 0 1 1 1 1
  spline S145 degree 3 poles (79.5484, 4.4881) (79.3452, 4.4058) (79.1486, 4.3292) (78.9588, 4.2579) knots 0 0 0 0 1 1 1 1
  arc A144 (78.9588, 4.2579) -> (78.7, 3.8638) centre (79.0995, 3.8835) ccw
  arc A145 (78.7606, 2.3228) -> (78.7, 3.8638) centre (0, 0) ccw
  arc A146 (78.7606, 2.3228) -> (79.0495, 1.9503) centre (79.1604, 2.3346) ccw
  spline S146 degree 3 poles (79.0495, 1.9503) (79.2443, 1.8941) (79.4462, 1.8331) (79.6553, 1.767) knots 0 0 0 0 1 1 1 1
  spline S147 degree 3 poles (79.6553, 1.767) (80.4293, 1.5221) (81.299, 1.2067) (82.2545, 0.8014) knots 0 0 0 0 1 1 1 1
  arc A147 (82.2545, -0.8014) -> (82.2545, 0.8014) centre (0, 0) ccw
  spline S148 degree 3 poles (82.2545, -0.8014) (81.299, -1.2067) (80.4293, -1.5221) (79.6553, -1.767) knots 0 0 0 0 1 1 1 1
  spline S149 degree 3 poles (79.6553, -1.767) (79.4462, -1.8331) (79.2443, -1.8941) (79.0495, -1.9503) knots 0 0 0 0 1 1 1 1
  arc A148 (79.0495, -1.9503) -> (78.7606, -2.3228) centre (79.1604, -2.3346) ccw
  arc A149 (78.7, -3.8638) -> (78.7606, -2.3228) centre (0, 0) ccw
  arc A150 (78.7, -3.8638) -> (78.9588, -4.2579) centre (79.0995, -3.8835) ccw
  spline S150 degree 3 poles (78.9588, -4.2579) (79.1486, -4.3292) (79.3452, -4.4058) (79.5484, -4.4881) knots 0 0 0 0 1 1 1 1
  spline S151 degree 3 poles (79.5484, -4.4881) (80.3008, -4.793) (81.1431, -5.1757) (82.0638, -5.6547) knots 0 0 0 0 1 1 1 1
  arc A151 (81.938, -7.2526) -> (82.0638, -5.6547) centre (0, 0) ccw
  spline S152 degree 3 poles (81.938, -7.2526) (80.9537, -7.5816) (80.0619, -7.8278) (79.2711, -8.0112) knots 0 0 0 0 1 1 1 1
  spline S153 degree 3 poles (79.2711, -8.0112) (79.0575, -8.0608) (78.8514, -8.1057) (78.6528, -8.1464) knots 0 0 0 0 1 1 1 1
  arc A152 (78.6528, -8.1464) -> (78.3355, -8.4951) centre (78.7332, -8.5383) ccw
  arc A153 (78.1543, -10.0267) -> (78.3355, -8.4951) centre (0, 0) ccw
  arc A154 (78.1543, -10.0267) -> (78.3813, -10.4398) centre (78.551, -10.0776) ccw
  spline S154 degree 3 poles (78.3813, -10.4398) (78.5649, -10.5258) (78.7549, -10.6176) (78.951, -10.7156) knots 0 0 0 0 1 1 1 1
  spline S155 degree 3 poles (78.951, -10.7156) (79.6772, -11.0785) (80.4868, -11.5261) (81.3672, -12.0759) knots 0 0 0 0 1 1 1 1
  arc A155 (81.1164, -13.659) -> (81.3672, -12.0759) centre (0, 0) ccw
  spline S156 degree 3 poles (81.1164, -13.659) (80.1093, -13.9098) (79.201, -14.0853) (78.3982, -14.2061) knots 0 0 0 0 1 1 1 1
  spline S157 degree 3 poles (78.3982, -14.2061) (78.1814, -14.2387) (77.9723, -14.2673) (77.7712, -14.2923) knots 0 0 0 0 1 1 1 1
  arc A156 (77.7712, -14.2923) -> (77.4275, -14.6151) centre (77.8206, -14.6893) ccw
  arc A157 (77.1267, -16.1277) -> (77.4275, -14.6151) centre (0, 0) ccw
  arc A158 (77.1267, -16.1277) -> (77.3206, -16.5573) centre (77.5182, -16.2095) ccw
  spline S158 degree 3 poles (77.3206, -16.5573) (77.4969, -16.6574) (77.6791, -16.7639) (77.8669, -16.877) knots 0 0 0 0 1 1 1 1
  spline S159 degree 3 poles (77.8669, -16.877) (78.5624, -17.2958) (79.3344, -17.8055) (80.1689, -18.4227) knots 0 0 0 0 1 1 1 1
  arc A159 (79.7947, -19.9812) -> (80.1689, -18.4227) centre (0, 0) ccw
  spline S160 degree 3 poles (79.7947, -19.9812) (78.771, -20.1522) (77.8517, -20.2559) (77.0419, -20.3133) knots 0 0 0 0 1 1 1 1
  spline S161 degree 3 poles (77.0419, -20.3133) (76.8232, -20.3288) (76.6126, -20.341) (76.41, -20.3501) knots 0 0 0 0 1 1 1 1
  arc A160 (76.41, -20.3501) -> (76.0422, -20.6449) centre (76.4282, -20.7497) ccw
  arc A161 (75.6235, -22.1292) -> (76.0422, -20.6449) centre (0, 0) ccw
  arc A162 (75.6235, -22.1292) -> (75.7832, -22.5728) centre (76.0074, -22.2416) ccw
  spline S162 degree 3 poles (75.7832, -22.5728) (75.9511, -22.6864) (76.1243, -22.8068) (76.3027, -22.9343) knots 0 0 0 0 1 1 1 1
  spline S163 degree 3 poles (76.3027, -22.9343) (76.9632, -23.4064) (77.6928, -23.9752) (78.4763, -24.6558) knots 0 0 0 0 1 1 1 1
  arc A163 (77.981, -26.1802) -> (78.4763, -24.6558) centre (0, 0) ccw
  spline S164 degree 3 poles (77.981, -26.1802) (76.9471, -26.2704) (76.0225, -26.3016) (75.2107, -26.2953) knots 0 0 0 0 1 1 1 1
  spline S165 degree 3 poles (75.2107, -26.2953) (74.9914, -26.2937) (74.7805, -26.2892) (74.5778, -26.2825) knots 0 0 0 0 1 1 1 1
  arc A164 (74.5778, -26.2825) -> (74.188, -26.5475) centre (74.5646, -26.6822) ccw
  arc A165 (73.6542, -27.9944) -> (74.188, -26.5475) centre (0, 0) ccw
  arc A166 (73.6542, -27.9944) -> (73.7785, -28.4491) centre (74.0281, -28.1365) ccw
  spline S166 degree 3 poles (73.7785, -28.4491) (73.937, -28.5755) (74.1003, -28.7092) (74.2681, -28.8503) knots 0 0 0 0 1 1 1 1
  spline S167 degree 3 poles (74.2681, -28.8503) (74.8895, -29.3727) (75.5723, -29.997) (76.2999, -30.737) knots 0 0 0 0 1 1 1 1
  arc A167 (75.6865, -32.2178) -> (76.2999, -30.737) centre (0, 0) ccw
  spline S168 degree 3 poles (75.6865, -32.2178) (74.6487, -32.2266) (73.7245, -32.1852) (72.9157, -32.1152) knots 0 0 0 0 1 1 1 1
  spline S169 degree 3 poles (72.9157, -32.1152) (72.6972, -32.0964) (72.4873, -32.0754) (72.2858, -32.0528) knots 0 0 0 0 1 1 1 1
  arc A168 (72.2858, -32.0528) -> (71.8764, -32.2864) centre (72.2413, -32.4503) ccw
  arc A169 (71.2307, -33.6869) -> (71.8764, -32.2864) centre (0, 0) ccw
  arc A170 (71.2307, -33.6869) -> (71.319, -34.15) centre (71.5923, -33.8579) ccw
  spline S170 degree 3 poles (71.319, -34.15) (71.4671, -34.2885) (71.6193, -34.4345) (71.7756, -34.5883) knots 0 0 0 0 1 1 1 1
  spline S171 degree 3 poles (71.7756, -34.5883) (72.3541, -35.1579) (72.9858, -35.8338) (73.6531, -36.6287) knots 0 0 0 0 1 1 1 1
  arc A171 (72.9254, -38.0568) -> (73.6531, -36.6287) centre (0, 0) ccw
  spline S172 degree 3 poles (72.9254, -38.0568) (71.8901, -37.9841) (70.972, -37.8704) (70.1712, -37.7371) knots 0 0 0 0 1 1 1 1
  spline S173 degree 3 poles (70.1712, -37.7371) (69.9549, -37.7012) (69.7473, -37.6638) (69.5482, -37.6254) knots 0 0 0 0 1 1 1 1
  arc A172 (69.5482, -37.6254) -> (69.1217, -37.8262) centre (69.4726, -38.0182) ccw
  arc A173 (68.3681, -39.1718) -> (69.1217, -37.8262) centre (0, 0) ccw
  arc A174 (68.3681, -39.1718) -> (68.4198, -39.6403) centre (68.7152, -39.3706) ccw
  spline S174 degree 3 poles (68.4198, -39.6403) (68.5565, -39.79) (68.6969, -39.9475) (68.8406, -40.1132) knots 0 0 0 0 1 1 1 1
  spline S175 degree 3 poles (68.8406, -40.1132) (69.3726, -40.7264) (69.9493, -41.4498) (70.5522, -42.2945) knots 0 0 0 0 1 1 1 1
  arc A175 (69.7147, -43.6612) -> (70.5522, -42.2945) centre (0, 0) ccw
  spline S176 degree 3 poles (69.7147, -43.6612) (68.6883, -43.5075) (67.7819, -43.322) (66.9941, -43.1264) knots 0 0 0 0 1 1 1 1
  spline S177 degree 3 poles (66.9941, -43.1264) (66.7812, -43.0736) (66.5772, -43.02) (66.3817, -42.9661) knots 0 0 0 0 1 1 1 1
  arc A176 (66.3817, -42.9661) -> (65.9408, -43.1328) centre (66.2755, -43.3518) ccw
  arc A177 (65.084, -44.4151) -> (65.9408, -43.1328) centre (0, 0) ccw
  arc A178 (65.084, -44.4151) -> (65.0987, -44.8863) centre (65.4144, -44.6406) ccw
  spline S178 degree 3 poles (65.0987, -44.8863) (65.2233, -45.0463) (65.3508, -45.2143) (65.4811, -45.3907) knots 0 0 0 0 1 1 1 1
  spline S179 degree 3 poles (65.4811, -45.3907) (65.9633, -46.0437) (66.4815, -46.8101) (67.0163, -47.6996) knots 0 0 0 0 1 1 1 1
  arc A179 (66.0742, -48.9963) -> (67.0163, -47.6996) centre (0, 0) ccw
  spline S180 degree 3 poles (66.0742, -48.9963) (65.063, -48.7626) (64.174, -48.5066) (63.4039, -48.2497) knots 0 0 0 0 1 1 1 1
  spline S181 degree 3 poles (63.4039, -48.2497) (63.1959, -48.1804) (62.9966, -48.111) (62.806, -48.0419) knots 0 0 0 0 1 1 1 1
  arc A180 (62.806, -48.0419) -> (62.3533, -48.1735) centre (62.6699, -48.418) ccw
  arc A181 (61.3986, -49.3846) -> (62.3533, -48.1735) centre (0, 0) ccw
  arc A182 (61.3986, -49.3846) -> (61.3763, -49.8555) centre (61.7102, -49.6353) ccw
  spline S182 degree 3 poles (61.3763, -49.8555) (61.4879, -50.0247) (61.6019, -50.2023) (61.7179, -50.3883) knots 0 0 0 0 1 1 1 1
  spline S183 degree 3 poles (61.7179, -50.3883) (62.1475, -51.0772) (62.6039, -51.8819) (63.0673, -52.8106) knots 0 0 0 0 1 1 1 1
  arc A183 (62.0263, -54.0294) -> (63.0673, -52.8106) centre (0, 0) ccw
  spline S184 degree 3 poles (62.0263, -54.0294) (61.0366, -53.717) (60.1704, -53.3921) (59.4228, -53.0756) knots 0 0 0 0 1 1 1 1
  spline S185 degree 3 poles (59.4228, -53.0756) (59.2209, -52.9901) (59.0277, -52.9053) (58.8431, -52.8215) knots 0 0 0 0 1 1 1 1
  arc A184 (58.8431, -52.8215) -> (58.3815, -52.9172) centre (58.6778, -53.1858) ccw
  arc A185 (57.3346, -54.0497) -> (58.3815, -52.9172) centre (0, 0) ccw
  arc A186 (57.3346, -54.0497) -> (57.2755, -54.5174) centre (57.6257, -54.324) ccw
  spline S186 degree 3 poles (57.2755, -54.5174) (57.3735, -54.6948) (57.4732, -54.8807) (57.5742, -55.0753) knots 0 0 0 0 1 1 1 1
  spline S187 degree 3 poles (57.5742, -55.0753) (57.9484, -55.7958) (58.3403, -56.6338) (58.7294, -57.596) knots 0 0 0 0 1 1 1 1
  arc A187 (57.596, -58.7294) -> (58.7294, -57.596) centre (0, 0) ccw
  spline S188 degree 3 poles (57.596, -58.7294) (56.6338, -58.3403) (55.7958, -57.9484) (55.0753, -57.5742) knots 0 0 0 0 1 1 1 1
  spline S189 degree 3 poles (55.0753, -57.5742) (54.8807, -57.4732) (54.6948, -57.3735) (54.5174, -57.2755) knots 0 0 0 0 1 1 1 1
  arc A188 (54.5174, -57.2755) -> (54.0497, -57.3346) centre (54.324, -57.6257) ccw
  arc A189 (52.9172, -58.3815) -> (54.0497, -57.3346) centre (0, 0) ccw
  arc A190 (52.9172, -58.3815) -> (52.8215, -58.8431) centre (53.1858, -58.6778) ccw
  spline S190 degree 3 poles (52.8215, -58.8431) (52.9053, -59.0277) (52.9901, -59.2209) (53.0756, -59.4228) knots 0 0 0 0 1 1 1 1
  spline S191 degree 3 poles (53.0756, -59.4228) (53.3921, -60.1704) (53.717, -61.0366) (54.0294, -62.0263) knots 0 0 0 0 1 1 1 1
  arc A191 (52.8106, -63.0673) -> (54.0294, -62.0263) centre (0, 0) ccw
  spline S192 degree 3 poles (52.8106, -63.0673) (51.8819, -62.6039) (51.0772, -62.1475) (50.3883, -61.7179) knots 0 0 0 0 1 1 1 1
  spline S193 degree 3 poles (50.3883, -61.7179) (50.2023, -61.6019) (50.0247, -61.4879) (49.8555, -61.3763) knots 0 0 0 0 1 1 1 1
  arc A192 (49.8555, -61.3763) -> (49.3846, -61.3986) centre (49.6353, -61.7102) ccw
  arc A193 (48.1735, -62.3533) -> (49.3846, -61.3986) centre (0, 0) ccw
  arc A194 (48.1735, -62.3533) -> (48.0419, -62.806) centre (48.418, -62.6699) ccw
  spline S194 degree 3 poles (48.0419, -62.806) (48.111, -62.9966) (48.1804, -63.1959) (48.2497, -63.4039) knots 0 0 0 0 1 1 1 1
  spline S195 degree 3 poles (48.2497, -63.4039) (48.5066, -64.174) (48.7626, -65.063) (48.9963, -66.0742) knots 0 0 0 0 1 1 1 1
  arc A195 (47.6996, -67.0163) -> (48.9963, -66.0742) centre (0, 0) ccw
  spline S196 degree 3 poles (47.6996, -67.0163) (46.8101, -66.4815) (46.0437, -65.9633) (45.3907, -65.4811) knots 0 0 0 0 1 1 1 1
  spline S197 degree 3 poles (45.3907, -65.4811) (45.2143, -65.3508) (45.0463, -65.2233) (44.8863, -65.0987) knots 0 0 0 0 1 1 1 1
  arc A196 (44.8863, -65.0987) -> (44.4151, -65.084) centre (44.6406, -65.4144) ccw
  arc A197 (43.1328, -65.9408) -> (44.4151, -65.084) centre (0, 0) ccw
  arc A198 (43.1328, -65.9408) -> (42.9661, -66.3817) centre (43.3518, -66.2755) ccw
  spline S198 degree 3 poles (42.9661, -66.3817) (43.02, -66.5772) (43.0736, -66.7812) (43.1264, -66.9941) knots 0 0 0 0 1 1 1 1
  spline S199 degree 3 poles (43.1264, -66.9941) (43.322, -67.7819) (43.5075, -68.6883) (43.6612, -69.7147) knots 0 0 0 0 1 1 1 1
  arc A199 (42.2945, -70.5522) -> (43.6612, -69.7147) centre (0, 0) ccw
  spline S200 degree 3 poles (42.2945, -70.5522) (41.4498, -69.9493) (40.7264, -69.3726) (40.1132, -68.8406) knots 0 0 0 0 1 1 1 1
  spline S201 degree 3 poles (40.1132, -68.8406) (39.9475, -68.6969) (39.79, -68.5565) (39.6403, -68.4198) knots 0 0 0 0 1 1 1 1
  arc A200 (39.6403, -68.4198) -> (39.1718, -68.3681) centre (39.3706, -68.7152) ccw
  arc A201 (37.8262, -69.1217) -> (39.1718, -68.3681) centre (0, 0) ccw
  arc A202 (37.8262, -69.1217) -> (37.6254, -69.5482) centre (38.0182, -69.4726) ccw